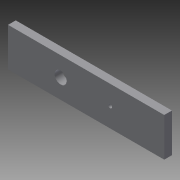
# Autodesk Inventor part: column
Saved by Autodesk Inventor 2016 (Build 200138000, 138)
## iProperties
Created: 2015-09-10
Part Number: column
Material: Wood (Oak)
Document SubType Name: Modeling
Designer: Students
Density: 0.76 g/cm^3
Appearance: White Oak - Natural Medium Gloss
Author: Students
Autodesk Inventor part; units mm, degrees
ref_plane "YZ Plane" through (0, 0, 0) normal (1, 0, 0) x (0, 1, 0)
ref_plane "XZ Plane" through (0, 0, 0) normal (0, 1, 0) x (-1, 0, 0)
ref_plane "XY Plane" through (0, 0, 0) normal (0, 0, 1) x (1, 0, 0)
sketch "Sketch1" plane through (0, 0, 0) normal (0, 1, 0) x (-1, 0, 0)
  line L0 (0, 0) -> (202, 0)
  line L1 (202, 0) -> (202, 50)
  line L2 (202, 50) -> (0, 50)
  line L3 (0, 50) -> (0, 0)
  circle A0 centre (70, 25) radius 2.5
  circle A1 centre (134, 25) radius 7.8
  constraints: 8 end point, 4 coincident, 2 centre point, 2 parallel, 1 horizontal, 1 perpendicular
extrude "Extrusion1" add sketch "Sketch1" along normal blind 10
body "Solid1"
